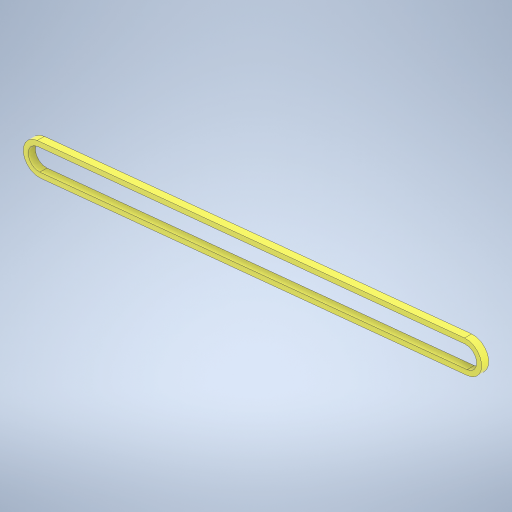
# Autodesk Inventor part: faja
Saved by Autodesk Inventor 2023 (Build 270158000, 158)
## iProperties
Created: 2022-04-05
Part Number: faja
Material: Genérico
Document SubType Name: Modeling
Designer: isaac
Density: 1 g/cm^3
Appearance: Valor por defecto
Author: isaac
Autodesk Inventor part; units mm, degrees
ref_plane "YZ Plane" through (0, 0, 0) normal (1, 0, 0) x (0, 1, 0)
ref_plane "XZ Plane" through (0, 0, 0) normal (0, 1, 0) x (-1, 0, 0)
ref_plane "XY Plane" through (0, 0, 0) normal (0, 0, 1) x (1, 0, 0)
sketch "Boceto1" plane through (0, 0, 0) normal (0, 0, 1) x (1, 0, 0)
  arc A0 (-303.9864, -15.0738) -> (-301.0136, -44.9262) centre (-302.5, -30) ccw
  arc A1 (301.4864, 15.0738) -> (298.5136, 44.9262) centre (300, 30) ccw
  line L0 (-303.9864, -15.0738) -> (298.5136, 44.9262)
  line L1 (301.4864, 15.0738) -> (-301.0136, -44.9262)
  line L2 (-361.4241, -13.7591) -> (297.8199, 51.8917)
  arc A2 (302.1801, 8.1083) -> (297.8199, 51.8917) centre (300, 30) ccw
  line L3 (302.1801, 8.1083) -> (-300.3199, -51.8917)
  arc A3 (-304.6801, -8.1083) -> (-300.3199, -51.8917) centre (-302.5, -30) ccw
  point P0 (0, 0)
  dimension "d0" = 30
  dimension "d1" = 30
  dimension "d2" = 300
  dimension "d3" = 302.5
  dimension "d4" = 30
  dimension "d5" = 30
  dimension "d6" = 7
  dimension "d8" = 7
  constraints: 9 point on circle, 8 end point, 6 tangent, 4 centre point, 2 concentric, 2 point on line, 1 parallel
  measures "d0" diameter of A1
  measures "d1" diameter of A0
  measures "d2" horizontal distance of point (0, 0) A1.centre
  measures "d3" horizontal distance of point (0, 0) A0.centre
  measures "d4" vertical distance of point (0, 0) A1.centre
  measures "d5" vertical distance of A0.centre point (0, 0)
  measures "d6" distance between parallel lines of L0 L2
  measures "d8" distance between parallel lines of L3 L1
extrude "Extrusión1" add sketch "Boceto1" along normal blind 10
